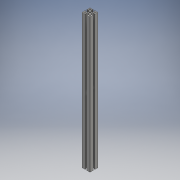
# Autodesk Inventor part: daeyoung_profile
Saved by Autodesk Inventor 2016 (Build 200138000, 138)
## iProperties
Created: 2024-05-31
Part Number: daeyoung_profile
Material: 일반
Document SubType Name: Modeling
Designer: pc
Density: 1 g/cm^3
Appearance: 기본값
Author: pc
Autodesk Inventor part; units mm, degrees
ref_plane "YZ Plane" through (0, 0, 0) normal (1, 0, 0) x (0, 1, 0)
ref_plane "XZ Plane" through (0, 0, 0) normal (0, 1, 0) x (-1, 0, 0)
ref_plane "XY Plane" through (0, 0, 0) normal (0, 0, 1) x (1, 0, 0)
sketch "스케치1" plane through (0, 0, 0) normal (0, 0, 1) x (1, 0, 0)
  line L0 (14.7, -3.15) -> (12.8, -3.15)
  arc A0 (12.8, -3.15) -> (12.5, -3.45) centre (12.8, -3.45) ccw
  line L1 (12.5, -3.45) -> (12.5, -4.85)
  arc A1 (12.2, -5.15) -> (12.5, -4.85) centre (12.2, -4.85) ccw
  line L2 (12.2, -5.15) -> (6.6786, -5.15)
  arc A2 (6.4569, -5.0521) -> (6.6786, -5.15) centre (6.6786, -4.85) ccw
  arc A3 (4.5043, -0.2543) -> (6.4569, -5.0521) centre (12, 0) ccw
  line L3 (4.5043, -0.2543) -> (4.25, 0)
  line L4 (4.25, 0) -> (4.5043, 0.2543)
  arc A4 (6.4569, 5.0521) -> (4.5043, 0.2543) centre (12, 0) ccw
  arc A5 (6.6786, 5.15) -> (6.4569, 5.0521) centre (6.6786, 4.85) ccw
  line L5 (6.6786, 5.15) -> (12.2, 5.15)
  arc A6 (12.5, 4.85) -> (12.2, 5.15) centre (12.2, 4.85) ccw
  line L6 (12.5, 4.85) -> (12.5, 3.45)
  arc A7 (12.5, 3.45) -> (12.8, 3.15) centre (12.8, 3.45) ccw
  line L7 (12.8, 3.15) -> (14.7, 3.15)
  arc A8 (14.7, 3.15) -> (15, 3.45) centre (14.7, 3.45) ccw
  line L8 (15, 3.45) -> (15, 14)
  arc A9 (15, 14) -> (14, 15) centre (14, 14) ccw
  line L9 (14, 15) -> (3.45, 15)
  arc A10 (3.45, 15) -> (3.15, 14.7) centre (3.45, 14.7) ccw
  line L10 (3.15, 14.7) -> (3.15, 12.8)
  arc A11 (3.15, 12.8) -> (3.45, 12.5) centre (3.45, 12.8) ccw
  line L11 (3.45, 12.5) -> (4.85, 12.5)
  arc A12 (5.15, 12.2) -> (4.85, 12.5) centre (4.85, 12.2) ccw
  line L12 (5.15, 12.2) -> (5.15, 6.6786)
  arc A13 (5.0521, 6.4569) -> (5.15, 6.6786) centre (4.85, 6.6786) ccw
  arc A14 (0.2543, 4.5043) -> (5.0521, 6.4569) centre (0, 12) ccw
  line L13 (0.2543, 4.5043) -> (0, 4.25)
  line L14 (0, 4.25) -> (-0.2543, 4.5043)
  arc A15 (-5.0521, 6.4569) -> (-0.2543, 4.5043) centre (0, 12) ccw
  arc A16 (-5.15, 6.6786) -> (-5.0521, 6.4569) centre (-4.85, 6.6786) ccw
  line L15 (-5.15, 6.6786) -> (-5.15, 12.2)
  arc A17 (-4.85, 12.5) -> (-5.15, 12.2) centre (-4.85, 12.2) ccw
  line L16 (-4.85, 12.5) -> (-3.45, 12.5)
  arc A18 (-3.45, 12.5) -> (-3.15, 12.8) centre (-3.45, 12.8) ccw
  line L17 (-3.15, 12.8) -> (-3.15, 14.7)
  arc A19 (-3.15, 14.7) -> (-3.45, 15) centre (-3.45, 14.7) ccw
  line L18 (-3.45, 15) -> (-14, 15)
  arc A20 (-14, 15) -> (-15, 14) centre (-14, 14) ccw
  line L19 (-15, 14) -> (-15, 3.45)
  arc A21 (-15, 3.45) -> (-14.7, 3.15) centre (-14.7, 3.45) ccw
  line L20 (-14.7, 3.15) -> (-12.8, 3.15)
  arc A22 (-12.8, 3.15) -> (-12.5, 3.45) centre (-12.8, 3.45) ccw
  line L21 (-12.5, 3.45) -> (-12.5, 4.85)
  arc A23 (-12.2, 5.15) -> (-12.5, 4.85) centre (-12.2, 4.85) ccw
  line L22 (-12.2, 5.15) -> (-6.6786, 5.15)
  arc A24 (-6.4569, 5.0521) -> (-6.6786, 5.15) centre (-6.6786, 4.85) ccw
  arc A25 (-4.5043, 0.2543) -> (-6.4569, 5.0521) centre (-12, 0) ccw
  line L23 (-4.5043, 0.2543) -> (-4.25, 0)
  line L24 (-4.25, 0) -> (-4.5043, -0.2543)
  arc A26 (-6.4569, -5.0521) -> (-4.5043, -0.2543) centre (-12, 0) ccw
  arc A27 (-6.6786, -5.15) -> (-6.4569, -5.0521) centre (-6.6786, -4.85) ccw
  line L25 (-6.6786, -5.15) -> (-12.2, -5.15)
  arc A28 (-12.5, -4.85) -> (-12.2, -5.15) centre (-12.2, -4.85) ccw
  line L26 (-12.5, -4.85) -> (-12.5, -3.45)
  arc A29 (-12.5, -3.45) -> (-12.8, -3.15) centre (-12.8, -3.45) ccw
  line L27 (-12.8, -3.15) -> (-14.7, -3.15)
  arc A30 (-14.7, -3.15) -> (-15, -3.45) centre (-14.7, -3.45) ccw
  line L28 (-15, -3.45) -> (-15, -14)
  arc A31 (-15, -14) -> (-14, -15) centre (-14, -14) ccw
  line L29 (-14, -15) -> (-3.45, -15)
  arc A32 (-3.45, -15) -> (-3.15, -14.7) centre (-3.45, -14.7) ccw
  line L30 (-3.15, -14.7) -> (-3.15, -12.8)
  arc A33 (-3.15, -12.8) -> (-3.45, -12.5) centre (-3.45, -12.8) ccw
  line L31 (-3.45, -12.5) -> (-4.85, -12.5)
  arc A34 (-5.15, -12.2) -> (-4.85, -12.5) centre (-4.85, -12.2) ccw
  line L32 (-5.15, -12.2) -> (-5.15, -6.6786)
  arc A35 (-5.0521, -6.4569) -> (-5.15, -6.6786) centre (-4.85, -6.6786) ccw
  arc A36 (-0.2543, -4.5043) -> (-5.0521, -6.4569) centre (0, -12) ccw
  line L33 (-0.2543, -4.5043) -> (0, -4.25)
  line L34 (0, -4.25) -> (0.2543, -4.5043)
  arc A37 (5.0521, -6.4569) -> (0.2543, -4.5043) centre (0, -12) ccw
  arc A38 (5.15, -6.6786) -> (5.0521, -6.4569) centre (4.85, -6.6786) ccw
  line L35 (5.15, -6.6786) -> (5.15, -12.2)
  arc A39 (4.85, -12.5) -> (5.15, -12.2) centre (4.85, -12.2) ccw
  line L36 (4.85, -12.5) -> (3.45, -12.5)
  arc A40 (3.45, -12.5) -> (3.15, -12.8) centre (3.45, -12.8) ccw
  line L37 (3.15, -12.8) -> (3.15, -14.7)
  arc A41 (3.15, -14.7) -> (3.45, -15) centre (3.45, -14.7) ccw
  line L38 (3.45, -15) -> (14, -15)
  arc A42 (14, -15) -> (15, -14) centre (14, -14) ccw
  line L39 (15, -14) -> (15, -3.45)
  arc A43 (15, -3.45) -> (14.7, -3.15) centre (14.7, -3.45) ccw
  arc A44 (-1.189, -2.1992) -> (1.189, -2.1992) centre (0, 0) ccw
  arc A45 (1.5438, -2.2509) -> (1.189, -2.1992) centre (1.3317, -2.4631) ccw
  line L40 (1.5438, -2.2509) -> (1.9092, -2.6163)
  arc A46 (1.9092, -2.6163) -> (2.3335, -2.6163) centre (2.1213, -2.4042) ccw
  line L41 (2.3335, -2.6163) -> (2.6163, -2.3335)
  arc A47 (2.6163, -2.3335) -> (2.6163, -1.9092) centre (2.4042, -2.1213) ccw
  line L42 (2.6163, -1.9092) -> (2.2509, -1.5438)
  arc A48 (2.1992, -1.189) -> (2.2509, -1.5438) centre (2.4631, -1.3317) ccw
  arc A49 (2.1992, -1.189) -> (2.1992, 1.189) centre (0, 0) ccw
  arc A50 (2.2509, 1.5438) -> (2.1992, 1.189) centre (2.4631, 1.3317) ccw
  line L43 (2.2509, 1.5438) -> (2.6163, 1.9092)
  arc A51 (2.6163, 1.9092) -> (2.6163, 2.3335) centre (2.4042, 2.1213) ccw
  line L44 (2.6163, 2.3335) -> (2.3335, 2.6163)
  arc A52 (2.3335, 2.6163) -> (1.9092, 2.6163) centre (2.1213, 2.4042) ccw
  line L45 (1.9092, 2.6163) -> (1.5438, 2.2509)
  arc A53 (1.189, 2.1992) -> (1.5438, 2.2509) centre (1.3317, 2.4631) ccw
  arc A54 (1.189, 2.1992) -> (-1.189, 2.1992) centre (0, 0) ccw
  arc A55 (-1.5438, 2.2509) -> (-1.189, 2.1992) centre (-1.3317, 2.4631) ccw
  line L46 (-1.5438, 2.2509) -> (-1.9092, 2.6163)
  arc A56 (-1.9092, 2.6163) -> (-2.3335, 2.6163) centre (-2.1213, 2.4042) ccw
  line L47 (-2.3335, 2.6163) -> (-2.6163, 2.3335)
  arc A57 (-2.6163, 2.3335) -> (-2.6163, 1.9092) centre (-2.4042, 2.1213) ccw
  line L48 (-2.6163, 1.9092) -> (-2.2509, 1.5438)
  arc A58 (-2.1992, 1.189) -> (-2.2509, 1.5438) centre (-2.4631, 1.3317) ccw
  arc A59 (-2.1992, 1.189) -> (-2.1992, -1.189) centre (0, 0) ccw
  arc A60 (-2.2509, -1.5438) -> (-2.1992, -1.189) centre (-2.4631, -1.3317) ccw
  line L49 (-2.2509, -1.5438) -> (-2.6163, -1.9092)
  arc A61 (-2.6163, -1.9092) -> (-2.6163, -2.3335) centre (-2.4042, -2.1213) ccw
  line L50 (-2.6163, -2.3335) -> (-2.3335, -2.6163)
  arc A62 (-2.3335, -2.6163) -> (-1.9092, -2.6163) centre (-2.1213, -2.4042) ccw
  line L51 (-1.9092, -2.6163) -> (-1.5438, -2.2509)
  arc A63 (-1.189, -2.1992) -> (-1.5438, -2.2509) centre (-1.3317, -2.4631) ccw
  circle A64 centre (10, -10) radius 3
  circle A65 centre (10, 10) radius 3
  circle A66 centre (-10, -10) radius 3
  circle A67 centre (-10, 10) radius 3
  point P0 (0, 0)
  constraints: 128 point on circle, 104 end point, 68 centre point
extrude "돌출1" add sketch "스케치1" along normal blind 500
